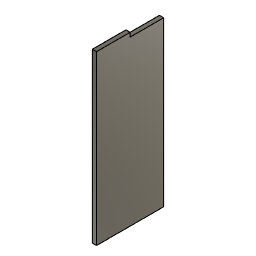
_ShelfShortSupport.ba8e0098-d5e9-4831-8ab2-3f400cf24f32 (Autodesk Fusion 360 design; units mm, degrees)
Autodesk Fusion 360 part; units mm, degrees
sketch "Sketch1" plane through (0, 0, 0) normal (1, 0, 0) x (0, 1, 0)
  line L0 (0, 0) -> (101.6, 0)
  line L1 (101.6, 0) -> (101.6, 254)
  line L2 (101.6, 254) -> (0, 254)
  line L3 (0, 254) -> (0, 0)
  line L4 (101.6, 254) -> (50.8, 254)
  line L5 (50.8, 254) -> (50.8, 247.65)
  line L6 (50.8, 247.65) -> (101.6, 247.65)
  line L7 (101.6, 247.65) -> (101.6, 254)
  dimension "d1" = 101.6
  dimension "d2" = 254
  dimension "d3" = 6.35
  dimension "d4" = 50.8
  constraint horizontal L0
  constraint vertical L1
  constraint horizontal L2
  constraint vertical L3
  constraint coincident L0.start L3.end
  constraint horizontal L4
  constraint vertical L5
  constraint horizontal L6
  constraint vertical L7
  constraint coincident L2 L1.end
  constraint collinear L1 L7
  measures "d1" distance of L0.start L0.end
  measures "d2" distance of L0.end L1.end
  measures "d3" distance of L4.end L5.end
  measures "d4" distance of L1 L5
extrude "Extrude1" add sketch "Sketch1" along normal blind 6.35 contours L0 L1 L2 L3 L5 L6
